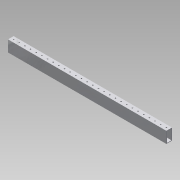
# Autodesk Inventor part: front rail
Saved by Autodesk Inventor 2015 (Build 190159000, 159)
## iProperties
Created: 2015-12-17
Part Number: front rail
Material: Aluminum 6061
Document SubType Name: Modeling
Designer: Daniel
Density: 2.7 g/cm^3
Appearance: Aluminum - Flat
Author: Daniel
Autodesk Inventor part; units mm, degrees
ref_plane "YZ Plane" through (0, 0, 0) normal (1, 0, 0) x (0, 1, 0)
ref_plane "XZ Plane" through (0, 0, 0) normal (0, 1, 0) x (-1, 0, 0)
ref_plane "XY Plane" through (0, 0, 0) normal (0, 0, 1) x (1, 0, 0)
sketch "Sketch1" plane through (0, 0, 0) normal (1, 0, 0) x (0, 1, 0)
  line L0 (0, 0) -> (50.8, 0)
  line L1 (50.8, 0) -> (50.8, -25.4)
  line L2 (50.8, -25.4) -> (0, -25.4)
  line L3 (0, -25.4) -> (0, 0)
  line L4 (48.26, -22.86) -> (48.26, -2.54)
  line L5 (48.26, -2.54) -> (2.54, -2.54)
  line L6 (2.54, -2.54) -> (2.54, -22.86)
  line L7 (2.54, -22.86) -> (48.26, -22.86)
  dimension "d0" = 50.8
  dimension "d1" = 25.4
  dimension "d2" = 2.54
  constraints: 16 end point, 4 parallel, 2 perpendicular, 1 horizontal, 3 other
  measures "d0" distance of L1.end L2.end
  measures "d1" distance of L0.end L1.end
  measures "d2" distance between parallel lines of L1 L4
extrude "Extrusion1" add sketch "Sketch1" along normal blind 711.2
sketch "Sketch3" plane through (0, 50.8, 0) normal (0, 1, 0) x (1, 0, 0)
  circle A0 centre (12.7, 12.7) radius 2.54
  line L0 (0, 0) -> (0, 25.4) projected
  line L1 (0, 0) -> (711.2, 0) projected
  dimension "d20" = 5.08
  dimension "d21" = 12.7
  dimension "d22" = 12.7
  constraints: 1 centre point
  measures "d20" diameter of A0
  measures "d21" distance from line of L0 A0.centre
  measures "d22" distance from line of L1 A0.centre
extrude "Extrusion3" cut sketch "Sketch3" against normal through all
pattern_linear "Rectangular Pattern1" count 28 spacing 25.4 along (1, 0, 0) of "Extrusion3"
body "Solid1"
